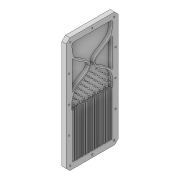
# Autodesk Inventor part: GB-mainsection
Saved by Autodesk Inventor 2020 (Build 240168000, 168)
## iProperties
Created: 2021-06-24
Part Number: GB-mainsection
Material: Generic
Document SubType Name: Modeling
Designer: Aidan Lee
Density: 1 g/cm^3
Appearance: Default
Author: Aidan Lee
Autodesk Inventor part; units mm, degrees
ref_plane "YZ Plane" through (0, 0, 0) normal (1, 0, 0) x (0, 1, 0)
ref_plane "XZ Plane" through (0, 0, 0) normal (0, 1, 0) x (-1, 0, 0)
ref_plane "XY Plane" through (0, 0, 0) normal (0, 0, 1) x (1, 0, 0)
sketch "Sketch1" plane through (0, 0, 0) normal (0, 0, 1) x (1, 0, 0)
  line L0 (0, 0) -> (140, 0)
  line L1 (140, 0) -> (140, 310)
  line L2 (140, 310) -> (0, 310)
  line L3 (0, 310) -> (0, 0)
  line L4 (15, 295) -> (125, 295) construction
  line L5 (125, 295) -> (125, 15) construction
  line L6 (125, 15) -> (15, 15) construction
  line L7 (15, 15) -> (15, 295) construction
  line L8 (15, 295) -> (125, 295) construction
  line L9 (70, 314.0975) -> (70, 322.6254) construction
  line L10 (15, 295) -> (15, 269.8596) construction
  line L11 (125, 295) -> (125, 292.6022) construction
  line L12 (0, 165.5) -> (-18, 165.5)
  line L13 (-18, 165.5) -> (-18, 185.5)
  line L14 (-18, 185.5) -> (0, 185.5) construction
  line L15 (0, 185.5) -> (0, 165.5)
  line L16 (-24.3067, 155) -> (-34.4998, 155) construction
  circle A0 centre (-9, 175.5) radius 3
  line L17 (-18, 185.5) -> (0, 205.5)
  line L18 (0, 144.5) -> (-18, 144.5)
  line L19 (-18, 144.5) -> (-18, 124.5)
  circle A1 centre (-9, 134.5) radius 3
  line L20 (-18, 124.5) -> (0, 104.5)
  line L21 (140, 165.5) -> (158, 165.5)
  line L22 (158, 165.5) -> (158, 185.5)
  circle A2 centre (149, 175.5) radius 3
  line L23 (158, 185.5) -> (140, 205.5)
  line L24 (158, 144.5) -> (158, 124.5)
  line L25 (140, 144.5) -> (158, 144.5)
  circle A3 centre (149, 134.5) radius 3
  line L26 (158, 124.5) -> (140, 104.5)
  line L27 (0, 300.2843) -> (9.7157, 310)
  line L28 (140, 300.2843) -> (130.2843, 310)
  line L29 (0, 9.7157) -> (9.7157, 0)
  line L30 (140, 9.7157) -> (130.2843, 0)
  line L31 (70, 295) -> (70, 310) construction
  line L32 (0, 155) -> (15, 155) construction
  line L33 (23.9173, 286.0827) -> (15, 295) construction
  line L34 (16.5096, 292.7523) -> (17.2477, 293.4904)
  line L35 (23.9173, 286.0827) -> (16.8787, 293.1213) construction
  line L36 (123.4904, 292.7523) -> (122.7523, 293.4904)
  line L37 (15, 17.2679) -> (15, 136.2679) construction
  line L38 (17, 136.2679) -> (17, 17.2679)
  arc A4 (17, 136.2679) -> (15, 136.2679) centre (16, 136.2679) ccw construction
  arc A5 (14, 16.2679) -> (15, 17.2679) centre (14, 17.2679) ccw construction
  line L39 (14, 16.2679) -> (12, 16.2679) construction
  arc A6 (17, 17.2679) -> (18, 16.2679) centre (18, 17.2679) ccw
  line L40 (20, 16.2679) -> (18, 16.2679)
  line L41 (21, 17.2679) -> (21, 136.2679)
  line L42 (23, 136.2679) -> (23, 17.2679)
  arc A7 (23, 17.2679) -> (24, 16.2679) centre (24, 17.2679) ccw
  arc A8 (23, 136.2679) -> (21, 136.2679) centre (22, 136.2679) ccw
  arc A9 (20, 16.2679) -> (21, 17.2679) centre (20, 17.2679) ccw
  line L43 (26, 16.2679) -> (24, 16.2679)
  line L44 (27, 17.2679) -> (27, 136.2679)
  line L45 (29, 136.2679) -> (29, 17.2679)
  arc A10 (29, 17.2679) -> (30, 16.2679) centre (30, 17.2679) ccw
  arc A11 (29, 136.2679) -> (27, 136.2679) centre (28, 136.2679) ccw
  arc A12 (26, 16.2679) -> (27, 17.2679) centre (26, 17.2679) ccw
  line L46 (32, 16.2679) -> (30, 16.2679)
  line L47 (33, 17.2679) -> (33, 136.2679)
  line L48 (35, 136.2679) -> (35, 17.2679)
  arc A13 (35, 17.2679) -> (36, 16.2679) centre (36, 17.2679) ccw
  arc A14 (35, 136.2679) -> (33, 136.2679) centre (34, 136.2679) ccw
  arc A15 (32, 16.2679) -> (33, 17.2679) centre (32, 17.2679) ccw
  line L49 (38, 16.2679) -> (36, 16.2679)
  line L50 (39, 17.2679) -> (39, 136.2679)
  line L51 (41, 136.2679) -> (41, 17.2679)
  arc A16 (41, 17.2679) -> (42, 16.2679) centre (42, 17.2679) ccw
  arc A17 (41, 136.2679) -> (39, 136.2679) centre (40, 136.2679) ccw
  arc A18 (38, 16.2679) -> (39, 17.2679) centre (38, 17.2679) ccw
  line L52 (44, 16.2679) -> (42, 16.2679)
  line L53 (45, 17.2679) -> (45, 136.2679)
  line L54 (47, 136.2679) -> (47, 17.2679)
  arc A19 (47, 17.2679) -> (48, 16.2679) centre (48, 17.2679) ccw
  arc A20 (47, 136.2679) -> (45, 136.2679) centre (46, 136.2679) ccw
  arc A21 (44, 16.2679) -> (45, 17.2679) centre (44, 17.2679) ccw
  line L55 (50, 16.2679) -> (48, 16.2679)
  line L56 (51, 17.2679) -> (51, 136.2679)
  line L57 (53, 136.2679) -> (53, 17.2679)
  arc A22 (53, 17.2679) -> (54, 16.2679) centre (54, 17.2679) ccw
  arc A23 (53, 136.2679) -> (51, 136.2679) centre (52, 136.2679) ccw
  arc A24 (50, 16.2679) -> (51, 17.2679) centre (50, 17.2679) ccw
  line L58 (56, 16.2679) -> (54, 16.2679)
  line L59 (57, 17.2679) -> (57, 136.2679)
  line L60 (59, 136.2679) -> (59, 17.2679)
  arc A25 (59, 17.2679) -> (60, 16.2679) centre (60, 17.2679) ccw
  arc A26 (59, 136.2679) -> (57, 136.2679) centre (58, 136.2679) ccw
  arc A27 (56, 16.2679) -> (57, 17.2679) centre (56, 17.2679) ccw
  line L61 (62, 16.2679) -> (60, 16.2679)
  line L62 (63, 17.2679) -> (63, 136.2679)
  line L63 (65, 136.2679) -> (65, 17.2679)
  arc A28 (65, 17.2679) -> (66, 16.2679) centre (66, 17.2679) ccw
  arc A29 (65, 136.2679) -> (63, 136.2679) centre (64, 136.2679) ccw
  arc A30 (62, 16.2679) -> (63, 17.2679) centre (62, 17.2679) ccw
  line L64 (68, 16.2679) -> (66, 16.2679)
  line L65 (69, 17.2679) -> (69, 136.2679)
  line L66 (71, 136.2679) -> (71, 17.2679)
  arc A31 (71, 17.2679) -> (72, 16.2679) centre (72, 17.2679) ccw
  arc A32 (71, 136.2679) -> (69, 136.2679) centre (70, 136.2679) ccw
  arc A33 (68, 16.2679) -> (69, 17.2679) centre (68, 17.2679) ccw
  line L67 (74, 16.2679) -> (72, 16.2679)
  line L68 (75, 17.2679) -> (75, 136.2679)
  line L69 (77, 136.2679) -> (77, 17.2679)
  arc A34 (77, 17.2679) -> (78, 16.2679) centre (78, 17.2679) ccw
  arc A35 (77, 136.2679) -> (75, 136.2679) centre (76, 136.2679) ccw
  arc A36 (74, 16.2679) -> (75, 17.2679) centre (74, 17.2679) ccw
  line L70 (80, 16.2679) -> (78, 16.2679)
  line L71 (81, 17.2679) -> (81, 136.2679)
  line L72 (83, 136.2679) -> (83, 17.2679)
  arc A37 (83, 17.2679) -> (84, 16.2679) centre (84, 17.2679) ccw
  arc A38 (83, 136.2679) -> (81, 136.2679) centre (82, 136.2679) ccw
  arc A39 (80, 16.2679) -> (81, 17.2679) centre (80, 17.2679) ccw
  line L73 (86, 16.2679) -> (84, 16.2679)
  line L74 (87, 17.2679) -> (87, 136.2679)
  line L75 (89, 136.2679) -> (89, 17.2679)
  arc A40 (89, 17.2679) -> (90, 16.2679) centre (90, 17.2679) ccw
  arc A41 (89, 136.2679) -> (87, 136.2679) centre (88, 136.2679) ccw
  arc A42 (86, 16.2679) -> (87, 17.2679) centre (86, 17.2679) ccw
  line L76 (92, 16.2679) -> (90, 16.2679)
  line L77 (93, 17.2679) -> (93, 136.2679)
  line L78 (95, 136.2679) -> (95, 17.2679)
  arc A43 (95, 17.2679) -> (96, 16.2679) centre (96, 17.2679) ccw
  arc A44 (95, 136.2679) -> (93, 136.2679) centre (94, 136.2679) ccw
  arc A45 (92, 16.2679) -> (93, 17.2679) centre (92, 17.2679) ccw
  line L79 (98, 16.2679) -> (96, 16.2679)
  line L80 (99, 17.2679) -> (99, 136.2679)
  line L81 (101, 136.2679) -> (101, 17.2679)
  arc A46 (101, 17.2679) -> (102, 16.2679) centre (102, 17.2679) ccw
  arc A47 (101, 136.2679) -> (99, 136.2679) centre (100, 136.2679) ccw
  arc A48 (98, 16.2679) -> (99, 17.2679) centre (98, 17.2679) ccw
  line L82 (104, 16.2679) -> (102, 16.2679)
  line L83 (105, 17.2679) -> (105, 136.2679)
  line L84 (107, 136.2679) -> (107, 17.2679)
  arc A49 (107, 17.2679) -> (108, 16.2679) centre (108, 17.2679) ccw
  arc A50 (107, 136.2679) -> (105, 136.2679) centre (106, 136.2679) ccw
  arc A51 (104, 16.2679) -> (105, 17.2679) centre (104, 17.2679) ccw
  line L85 (110, 16.2679) -> (108, 16.2679)
  line L86 (111, 17.2679) -> (111, 136.2679)
  line L87 (113, 136.2679) -> (113, 17.2679)
  arc A52 (113, 17.2679) -> (114, 16.2679) centre (114, 17.2679) ccw
  arc A53 (113, 136.2679) -> (111, 136.2679) centre (112, 136.2679) ccw
  arc A54 (110, 16.2679) -> (111, 17.2679) centre (110, 17.2679) ccw
  line L88 (116, 16.2679) -> (114, 16.2679)
  line L89 (117, 17.2679) -> (117, 136.2679)
  line L90 (119, 136.2679) -> (119, 17.2679)
  arc A55 (119, 17.2679) -> (120, 16.2679) centre (120, 17.2679) ccw
  arc A56 (119, 136.2679) -> (117, 136.2679) centre (118, 136.2679) ccw
  arc A57 (116, 16.2679) -> (117, 17.2679) centre (116, 17.2679) ccw
  line L91 (122, 16.2679) -> (120, 16.2679)
  line L92 (123, 17.2679) -> (123, 136.2679)
  line L93 (125, 136.2679) -> (125, 17.2679) construction
  arc A58 (125, 17.2679) -> (126, 16.2679) centre (126, 17.2679) ccw construction
  arc A59 (125, 136.2679) -> (123, 136.2679) centre (124, 136.2679) ccw construction
  arc A60 (122, 16.2679) -> (123, 17.2679) centre (122, 17.2679) ccw
  spline S0 degree 4 poles (16.5096, 292.7523) (14.6703, 290.9129) (15.6874, 287.8803) (14.9514, 263.0684) (27.2259, 252.1032) (45.0884, 239.248) (54.8331, 236.5084) (66.6786, 222.7415) (65.5, 220.3383) (65.5, 218.384) knots 0 0 0 0 0 0.198302 0.355061 0.529019 0.693641 0.832065 1 1 1 1 1
  line L94 (65.5, 218.384) -> (65.5, 202.0117) construction
  line L95 (74.5, 218.384) -> (74.5, 202.0117) construction
  spline S1 degree 4 poles (123.4904, 292.7523) (125.3297, 290.9129) (124.3126, 287.8803) (125.0486, 263.0684) (112.7741, 252.1032) (94.9116, 239.248) (85.1669, 236.5084) (73.3214, 222.7415) (74.5, 220.3383) (74.5, 218.384) knots 0 0 0 0 0 0.198302 0.355061 0.529019 0.693641 0.832065 1 1 1 1 1
  line L96 (65.5, 218.384) -> (74.5, 218.384) construction
  line L97 (65.5389, 141.7679) -> (74.4611, 141.7679) construction
  line L98 (70, 141.7679) -> (70, 218.384) construction
  line L99 (70, 218.384) -> (70, 295) construction
  line L100 (65.5, 218.384) -> (15, 218.384) construction
  line L101 (62.8466, 226.2847) -> (62.8466, 218.384) construction
  line L102 (57.0465, 232.5428) -> (57.0465, 218.384) construction
  line L103 (45.5, 240.1042) -> (45.5, 218.384) construction
  line L104 (28.8522, 251.4195) -> (28.8522, 218.384) construction
  line L105 (17.5, 267.9145) -> (17.5, 218.384) construction
  line L106 (15.2393, 288.9289) -> (15.2393, 218.384) construction
  spline S2 degree 4 poles (65.5, 218.384) (65.5, 215.0113) (62.762, 209.2142) (57.6098, 203.6988) (43.4805, 195.4527) (24.4915, 184.5352) (15.1033, 169.2275) (15, 156.1972) (15, 148.5289) knots 0 0 0 0 0 0.197939 0.350153 0.51962 0.706517 1 1 1 1 1
  line L107 (62.8466, 218.384) -> (62.8466, 210.4833) construction
  line L108 (57.0465, 218.384) -> (57.0465, 204.2251) construction
  line L109 (45.5, 218.384) -> (45.5, 196.6637) construction
  line L110 (28.8522, 218.384) -> (28.8522, 185.3485) construction
  line L111 (17.5, 218.384) -> (17.5, 168.8535) construction
  spline S3 degree 4 poles (74.5, 218.384) (74.5, 215.0113) (77.238, 209.2142) (82.3902, 203.6988) (96.5195, 195.4527) (115.5085, 184.5352) (124.8967, 169.2275) (125, 156.1972) (125, 148.5289) knots 0 0 0 0 0 0.197939 0.350153 0.51962 0.706517 1 1 1 1 1
  line L112 (125, 148.5289) -> (125, 140.8711) construction
  circle A61 centre (70, 198.7679) radius 1
  circle A62 centre (70, 184.7679) radius 1
  circle A63 centre (70, 170.7679) radius 1
  circle A64 centre (70, 156.7679) radius 1
  circle A65 centre (70, 142.7679) radius 1
  line L113 (-110.1015, 148.4668) -> (-137.337, 121.2312) construction
  line L114 (-137.337, 121.2312) -> (-99.9418, 121.2312) construction
  circle A66 centre (63, 191.7679) radius 1
  line L115 (209.7417, 198.7679) -> (209.7417, 184.7679) construction
  line L116 (63, 191.7679) -> (70, 198.7679) construction
  circle A67 centre (63, 177.7679) radius 1
  circle A68 centre (63, 163.7679) radius 1
  circle A69 centre (63, 149.7679) radius 1
  line L117 (70, 184.7679) -> (70, 170.7679) construction
  line L118 (70, 170.7679) -> (70, 156.7679) construction
  line L119 (70, 156.7679) -> (70, 142.7679) construction
  line L120 (63, 191.7679) -> (56, 184.7679) construction
  line L121 (56, 184.7679) -> (49, 177.7679) construction
  line L122 (49, 177.7679) -> (42, 170.7679) construction
  line L123 (42, 170.7679) -> (35, 163.7679) construction
  line L124 (35, 163.7679) -> (28, 156.7679) construction
  line L125 (28, 156.7679) -> (21, 149.7679) construction
  line L126 (21, 149.7679) -> (14, 142.7679) construction
  line L127 (14, 156.7679) -> (21, 163.7679) construction
  line L128 (21, 163.7679) -> (28, 170.7679) construction
  line L129 (28, 170.7679) -> (35.279, 178.047) construction
  line L130 (35.279, 178.047) -> (42, 184.7679) construction
  circle A70 centre (56, 184.7679) radius 1
  circle A71 centre (49, 177.7679) radius 1
  circle A72 centre (42, 184.7679) radius 1
  circle A73 centre (42, 170.7679) radius 1
  circle A74 centre (35, 177.7679) radius 1
  circle A75 centre (28, 170.7679) radius 1
  circle A76 centre (35, 163.7679) radius 1
  circle A77 centre (49, 163.7679) radius 1
  circle A78 centre (56, 170.7679) radius 1
  circle A79 centre (21, 163.7679) radius 1
  circle A80 centre (21, 149.7679) radius 1
  circle A81 centre (49, 191.7679) radius 1
  circle A82 centre (42, 156.7679) radius 1
  circle A83 centre (28, 156.7679) radius 1
  circle A84 centre (28, 142.7679) radius 1
  circle A85 centre (35, 149.7679) radius 1
  circle A86 centre (42, 142.7679) radius 1
  circle A87 centre (49, 149.7679) radius 1
  circle A88 centre (56, 156.7679) radius 1
  circle A89 centre (56, 142.7679) radius 1
  circle A90 centre (77, 191.7679) radius 1
  circle A91 centre (77, 177.7679) radius 1
  circle A92 centre (77, 163.7679) radius 1
  circle A93 centre (77, 149.7679) radius 1
  circle A94 centre (84, 184.7679) radius 1
  circle A95 centre (91, 177.7679) radius 1
  circle A96 centre (98, 184.7679) radius 1
  circle A97 centre (98, 170.7679) radius 1
  circle A98 centre (105, 177.7679) radius 1
  circle A99 centre (112, 170.7679) radius 1
  circle A100 centre (105, 163.7679) radius 1
  circle A101 centre (91, 163.7679) radius 1
  circle A102 centre (84, 170.7679) radius 1
  circle A103 centre (119, 163.7679) radius 1
  circle A104 centre (119, 149.7679) radius 1
  circle A105 centre (91, 191.7679) radius 1
  circle A106 centre (98, 156.7679) radius 1
  circle A107 centre (112, 156.7679) radius 1
  circle A108 centre (112, 142.7679) radius 1
  circle A109 centre (105, 149.7679) radius 1
  circle A110 centre (98, 142.7679) radius 1
  circle A111 centre (91, 149.7679) radius 1
  circle A112 centre (84, 156.7679) radius 1
  circle A113 centre (84, 142.7679) radius 1
  line L131 (15, 148.5289) -> (15, 140.2675)
  line L132 (125, 148.5289) -> (125, 140.2675)
  spline S4 degree 4 poles (17.2477, 293.4904) (18.1955, 294.4381) (19.6714, 295.0826) (20.7017, 295) (21.8623, 295) knots 0 0 0 0 0 1 1 1 1 1
  spline S5 degree 3 poles (122.7523, 293.4904) (121.4886, 294.7541) (119.4432, 295.1927) (118.1377, 295) knots 0 0 0 0 1 1 1 1
  line L133 (118.1377, 295) -> (21.8623, 295)
  line L134 (16.8787, 293.1213) -> (23.2316, 286.7684) construction
  arc A114 (19, 310) -> (0, 291) centre (19, 291) ccw construction
  arc A115 (19, 295) -> (15, 291) centre (19, 291) ccw construction
  line L135 (19, 291) -> (10, 291) construction
  line L136 (19, 291) -> (19, 300) construction
  line L137 (16.1716, 293.8284) -> (5.565, 304.435) construction
  circle A116 centre (10.8683, 299.1317) radius 2
  line L138 (9.8231, 300.915) -> (9.085, 300.1769) construction
  line L139 (11.9134, 297.3485) -> (12.6515, 298.0866) construction
  circle A117 centre (70, 302.5) radius 2
  circle A118 centre (7.5, 155) radius 2
  circle A119 centre (7.5, 227.0659) radius 2
  line L140 (7.5, 155) -> (7.5, 227.0659) construction
  line L141 (7.5, 227.0659) -> (7.5, 299.1317) construction
  arc A120 (140, 291) -> (121, 310) centre (121, 291) ccw construction
  arc A121 (125, 291) -> (121, 295) centre (121, 291) ccw construction
  circle A122 centre (129.1317, 299.1317) radius 2
  circle A123 centre (132.5, 155) radius 2
  circle A124 centre (132.5, 227.0659) radius 2
  circle A125 centre (10.8683, 10.8683) radius 2
  circle A126 centre (70, 7.5) radius 2
  circle A127 centre (7.5, 82.9341) radius 2
  circle A128 centre (132.5, 82.9341) radius 2
  circle A129 centre (129.1317, 10.8683) radius 2
  arc A130 (0, 19) -> (19, 0) centre (19, 19) ccw construction
  arc A131 (15, 19) -> (19, 15) centre (19, 19) ccw construction
  arc A132 (121, 0) -> (140, 19) centre (121, 19) ccw construction
  arc A133 (121, 15) -> (125, 19) centre (121, 19) ccw construction
  circle A134 centre (10.8683, 299.1317) radius 7.5 construction
  line L142 (4.4716, 303.3416) -> (6.8718, 305.7419) construction
  line L143 (15, 140.2675) -> (15, 136.2679) construction
  line L144 (123.2929, 136.9751) -> (125, 138.6822)
  arc A135 (123.2929, 136.9751) -> (123, 136.2679) centre (124, 136.2679) ccw
  line L145 (125, 138.6822) -> (125, 140.2675)
  line L146 (15, 138.6822) -> (16.7071, 136.9751)
  arc A136 (17, 136.2679) -> (16.7071, 136.9751) centre (16, 136.2679) ccw
  line L147 (15, 138.6822) -> (15, 140.2675)
  point P0 (70, 318.3615)
  point P1 (-29.4032, 155)
  point P2 (-18, 175.5)
  point P3 (-9, 185.5)
  point P4 (65.2876, 221.8871)
  point P5 (122.5, 267.9145)
  point P6 (111.1478, 251.4195)
  point P7 (94.5, 240.1042)
  point P8 (82.9535, 232.5428)
  point P9 (74.7124, 221.8871)
  point P10 (124.7607, 288.9289)
  point P11 (77.1534, 210.4833)
  point P12 (82.9535, 204.2251)
  point P13 (94.5, 196.6637)
  point P14 (111.1478, 185.3485)
  point P15 (122.5, 168.8535)
  point P16 (209.7417, 191.7679)
  point P17 (70, 177.7679)
  point P18 (70, 163.7679)
  point P19 (70, 149.7679)
  point P20 (19.6961, 294.835)
  point P21 (120.3039, 294.835)
  point P22 (9.4541, 300.5459)
  point P23 (12.2825, 297.7175)
  dimension "d163" = 4
  dimension "d0" = 140
  dimension "d1" = 310
  dimension "d2" = 15
  dimension "d85" = 18
  dimension "d86" = 20
  dimension "d87" = 10.5
  dimension "d88" = 6
  dimension "d89" = 20
  dimension "d114" = 135
  dimension "d124" = 2
  dimension "d126" = 1
  dimension "d128" = 2
  dimension "d136" = 6
  dimension "d141" = 9
  dimension "d142" = 5.5
  dimension "pegd" = 2
  dimension "d147" = 14
  dimension "d152" = 45
  dimension "d158" = 45
  dimension "d161" = 4
  dimension "d164" = 5.5
  dimension "d168" = 15
  dimension "d169" = 1
  dimension "d170" = 1
  dimension "d171" = 1
  dimension "d172" = 120
  dimension "d178" = 45
  dimension "d179" = 45
  constraints: 296 end point, 157 point on circle, 136 centre point, 85 symmetric about line, 47 point on line, 33 horizontal alignment, 25 equal radius, 24 vertical alignment, 21 midpoint, 18 vertical, 15 equal length, 14 coincident, 14 perpendicular, 13 collinear, 13 parallel, 12 horizontal, 9 tangent, 403 other
  measures "d0" distance of L0.start L0.end
  measures "d1" distance of L2.end L0.start
  measures "d2" distance between parallel lines of L2 L4
  measures "d85" distance of L13.end L14.end
  measures "d86" distance of L12.end L13.end
  measures "d87" distance between parallel lines of L12 L16
  measures "d88" diameter of A0
  measures "d89" vertical distance of L13.end L17.end
  measures "d114" angle of L3 L27
  measures "d124" distance between parallel lines of L37 L38
  measures "d126" radius of A5
  measures "d128" distance of L39.start L39.end
  measures "d136" distance of L39.start L40.start
  measures "d141" distance between parallel lines of L95 L94
  measures "d142" distance from line of A32.centre L97
  measures "pegd" diameter of A61
  measures "d147" distance of L116.end L117.start
  measures "d152" angle of L114 L113
  measures "d158" angle of L4 L35
  measures "d161" radius of A115
  measures "d164" distance edge to line of A114 L138
  measures "d168" diameter of A134
  measures "d169" distance between parallel lines of L27 L142
  measures "d170" distance from line of L137.start L34
  measures "d171" horizontal distance between centres of A131 A6
  measures "d172" distance from line of L40 A4.centre
  measures "d178" angle of L5 L144
  measures "d179" angle of L143 L146
extrude "Extrusion3" add sketch "Sketch1" against normal blind 2 contours L29 L3 L27 L2 L28 L1 L30 L0 | L34 S4 L133 S5 L36 S1 S3 L132 L145 L144 A135 L92 A60 L91 A55 L90 A56 L89 A57 L88 A52 L87 A53 L86 A54 L85 A49 L84 A50 L83 A51 L82 A46 L81 A47 L80 A48 L79 A43 L78 A44 L77 A45 L76 A40 L75 A41 L74 A42 L73 A37 L72 A38 L71 A39 L70 A34 L69 A35 L68 A36 L67 A31 L66 A32 L65 A33 L64 A28 L63 A29 L62 A30 L61 A25 L60 A26 L59 A27 L58 A22 L57 A23 L56 A24 L55 A19 L54 A20 L53 A21 L52 A16 L51 A17 L50 A18 L49 A13 L48 A14 L47 A15 L46 A10 L45 A11 L44 A12 L43 A7 L42 A8 L41 A9 L40 A6 L38 A136 L146 L147 L131 S2 S0 | A61 | A62 | A63 | A64 | A65 | A66 | A67 | A68 | A69 | A70 | A71 | A72 | A73 | A74 | A75 | A76 | A77 | A78 | A79 | A80 | A81 | A82 | A83 | A84 | A85 | A86 | A87 | A88 | A89 | A90 | A91 | A92 | A93 | A94 | A95 | A96 | A97 | A98 | A99 | A100 | A101 | A102 | A103 | A104 | A105 | A106 | A107 | A108 | A109 | A110 | A111 | A112 | A113
extrude "Extrusion4" add sketch "Sketch1" along normal blind 10 contours L29 L3 L27 L2 L28 L1 L30 L0 | A61 | A62 | A63 | A64 | A65 | A66 | A67 | A68 | A69 | A70 | A71 | A72 | A73 | A74 | A75 | A76 | A77 | A78 | A79 | A80 | A81 | A82 | A83 | A84 | A85 | A86 | A87 | A88 | A89 | A90 | A91 | A92 | A93 | A94 | A95 | A96 | A97 | A98 | A99 | A100 | A101 | A102 | A103 | A104 | A105 | A106 | A107 | A108 | A109 | A110 | A111 | A112 | A113
fillet "Fillet1" radius 1 53 edges at (83, 156.7679, 0) (20, 163.7679, 0) (34, 163.7679, 0) (27, 156.7679, 0) (48, 163.7679, 0) (48, 149.7679, 0) (34, 149.7679, 0) (20, 149.7679, 0) (62, 149.7679, 0) (55, 156.7679, 0) (76, 163.7679, 0) (111, 156.7679, 0) (69, 156.7679, 0) (41, 156.7679, 0) (62, 163.7679, 0) (76, 149.7679, 0) (97, 156.7679, 0) (104, 163.7679, 0) (90, 163.7679, 0) (104, 149.7679, 0) (118, 149.7679, 0) (90, 149.7679, 0) (118, 163.7679, 0) (41, 142.7679, 0) (55, 142.7679, 0) (69, 142.7679, 0) (83, 142.7679, 0) (27, 142.7679, 0) (111, 142.7679, 0) (97, 142.7679, 0) (48, 177.7679, 0) (27, 170.7679, 0) (55, 170.7679, 0) (76, 177.7679, 0) (90, 177.7679, 0) (41, 170.7679, 0) (34, 177.7679, 0) (62, 177.7679, 0) (69, 170.7679, 0) (97, 170.7679, 0) (104, 177.7679, 0) (111, 170.7679, 0) (83, 170.7679, 0) (83, 184.7679, 0) (97, 184.7679, 0) (41, 184.7679, 0) (55, 184.7679, 0) (69, 184.7679, 0) (90, 191.7679, 0) (62, 191.7679, 0) (48, 191.7679, 0) (76, 191.7679, 0) (69, 198.7679, 0)
sketch "Sketch2" plane through (0, 0, 10) normal (0, 0, 1) x (1, 0, 0)
  line L0 (124, 262.6757) -> (124, 174.0922)
  line L1 (140, 9.7157) -> (140, 300.2843) projected
  line L2 (77.5, 222.1577) -> (77.5, 214.6103) construction
  spline S0 degree 4 poles (77.5, 218.384) (77.5, 221.3006) (79.4995, 225.4222) (87.0228, 232.0065) (96.9122, 236.9983) (108.3676, 245.0298) (118.246, 251.5404) (121.4024, 256.862) (124, 262.6757) knots 0 0 0 0 0 0.204474 0.349165 0.501134 0.648623 1 1 1 1 1
  line L3 (65.5, 218.384) -> (74.5, 218.384) construction
  spline S1 degree 4 poles (77.5, 218.384) (77.5, 215.4673) (79.4995, 211.3458) (87.0228, 204.7614) (96.9122, 199.7696) (108.3676, 191.7382) (118.246, 185.2276) (121.4024, 179.906) (124, 174.0922) knots 0 0 0 0 0 0.204474 0.349165 0.501134 0.648623 1 1 1 1 1
  arc A0 (124, 255.8207) -> (120.9487, 256.7907) centre (122.3202, 255.8207) ccw
  arc A1 (120.9487, 179.9772) -> (124, 180.9473) centre (122.3202, 180.9473) ccw
  line L4 (70, 295) -> (70, 310) construction
  line L5 (16, 262.6757) -> (16, 174.0922)
  spline S2 degree 4 poles (62.5, 218.384) (62.9419, 222.6663) (56.3652, 230.3575) (45.9791, 235.0178) (31.6608, 244.9849) (21.7353, 251.57) (18.6069, 256.8473) (16, 262.6757) knots 0 0 0 0 0 0.349165 0.501134 0.648623 1 1 1 1 1
  spline S3 degree 4 poles (62.5, 218.384) (62.9419, 214.1016) (56.3652, 206.4105) (45.9791, 201.7502) (31.6608, 191.7831) (21.7353, 185.1979) (18.6069, 179.9207) (16, 174.0922) knots 0 0 0 0 0 0.349165 0.501134 0.648623 1 1 1 1 1
  arc A2 (19.0513, 256.7907) -> (16, 255.8207) centre (17.6798, 255.8207) ccw
  arc A3 (16, 180.9473) -> (19.0513, 179.9772) centre (17.6798, 180.9473) ccw
  point P0 (0, 0)
  point P1 (124, 218.384)
  point P2 (79.836, 224.6495)
  point P3 (87.5499, 231.6115)
  point P4 (96.7859, 237.2648)
  point P5 (105.7809, 243.1688)
  point P6 (114.0942, 249.2408)
  point P7 (119.7282, 255.0138)
  point P8 (79.836, 212.1185)
  point P9 (87.5499, 205.1564)
  point P10 (96.7859, 199.5031)
  point P11 (105.7809, 193.5991)
  point P12 (114.0942, 187.5272)
  point P13 (119.7282, 181.7542)
  point P14 (60.164, 224.6495)
  point P15 (52.4501, 231.6115)
  point P16 (43.2141, 237.2648)
  point P17 (34.2191, 243.1688)
  point P18 (25.9058, 249.2408)
  point P19 (20.2718, 255.0138)
  point P20 (60.164, 212.1185)
  point P21 (52.4501, 205.1564)
  point P22 (43.2141, 199.5031)
  point P23 (34.2191, 193.5991)
  point P24 (25.9058, 187.5272)
  point P25 (20.2718, 181.7542)
  point P26 (120.9487, 179.9772)
  point P27 (124, 180.9473)
  point P28 (16, 180.9473)
  point P29 (19.0513, 179.9772)
  dimension "d185" = 16
  dimension "d186" = 3
  constraints: 30 symmetric about line, 8 point on circle, 6 end point, 4 centre point, 3 vertical, 2 horizontal alignment, 2 midpoint, 2 point on line, 1 parallel, 1 tangent, 37 other
  measures "d185" distance between parallel lines of L1 L0
  measures "d186" distance from line of point (74.5, 218.384) L2
extrude "Extrusion5" cut sketch "Sketch2" against normal blind 10 contours L0 A1 S1 S0 A0 | A2 S2 S3 A3 L5
extrude "Extrusion6" add sketch "Sketch1" against normal mid plane 4 contours A116 | A117 | A118 | A119 | A122 | A123 | A124 | A125 | A126 | A127 | A128 | A129
thread "Thread1" size "M4x0.7" class "6H" standard "ANSI Metric M Profile" full length
thread "Thread2" size "M4x0.7" class "6H" standard "ANSI Metric M Profile" full length
thread "Thread3" size "M4x0.7" class "6H" standard "ANSI Metric M Profile" full length
thread "Thread4" size "M4x0.7" class "6H" standard "ANSI Metric M Profile" full length
thread "Thread5" size "M4x0.7" class "6H" standard "ANSI Metric M Profile" full length
thread "Thread6" size "M4x0.7" class "6H" standard "ANSI Metric M Profile" full length
thread "Thread7" size "M4x0.7" class "6H" standard "ANSI Metric M Profile" full length
thread "Thread8" size "M4x0.7" class "6H" standard "ANSI Metric M Profile" full length
thread "Thread9" size "M4x0.7" class "6H" standard "ANSI Metric M Profile" full length
thread "Thread10" size "M4x0.7" class "6H" standard "ANSI Metric M Profile" full length
thread "Thread11" size "M4x0.7" class "6H" standard "ANSI Metric M Profile" full length
thread "Thread12" size "M4x0.7" class "6H" standard "ANSI Metric M Profile" full length
sketch "Sketch3" plane through (0, 0, -2) normal (0, 0, -1) x (-1, 0, 0)
  circle A0 centre (-132.5, 155) radius 2 projected
  circle A1 centre (-132.5, 175) radius 3
  line L0 (24.3067, 155) -> (34.4998, 155) construction
  line L1 (-132.5, 155) -> (-119.86, 155)
  circle A2 centre (-132.5, 135) radius 3
  line L2 (-132.5, 175) -> (-119.86, 175) construction
  line L3 (-9.7157, 0) -> (-130.2843, 0) projected
  line L4 (-70, 0) -> (-70, 3.7209)
  circle A3 centre (-7.5, 175) radius 3
  circle A4 centre (-7.5, 135) radius 3
  point P0 (0, 0)
  dimension "d215" = 6
  dimension "d216" = 40
  constraints: 6 end point, 4 centre point, 3 symmetric about line, 2 horizontal, 1 midpoint, 1 vertical, 1 vertical alignment, 3 other
  measures "d215" diameter of A1
  measures "d216" diameter of L2 L1
extrude "Extrusion7" cut sketch "Sketch3" against normal blind 8 contours A1 | A2 | A3 | A4
thread "Thread13" size "M6x1" class "6H" standard "ANSI Metric M Profile" full length
thread "Thread14" size "M6x1" class "6H" standard "ANSI Metric M Profile" full length
thread "Thread15" size "M6x1" class "6H" standard "ANSI Metric M Profile" full length
thread "Thread16" size "M6x1" class "6H" standard "ANSI Metric M Profile" full length
body "Solid2"
